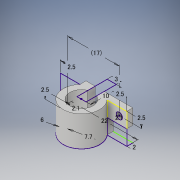
# Autodesk Inventor part: Ω型
Saved by Autodesk Inventor 2019.3 (Build 233278000, 278)
## iProperties
Created: 2019-08-08
Part Number: Ω型
Material: 一般
Document SubType Name: Modeling
Designer: naito
Density: 1 g/cm^3
Appearance: 既定
Author: naito
Autodesk Inventor part; units mm, degrees
ref_plane "YZ Plane" through (0, 0, 0) normal (1, 0, 0) x (0, 1, 0)
ref_plane "XZ Plane" through (0, 0, 0) normal (0, 1, 0) x (-1, 0, 0)
ref_plane "XY Plane" through (0, 0, 0) normal (0, 0, 1) x (1, 0, 0)
sketch "スケッチ3" plane through (0, 0, 0) normal (0, 1, 0) x (-1, 0, 0)
  circle A0 centre (0, 0) radius 3.85
  line L0 (11, -4) -> (4.4721, -4)
  line L1 (-11, -4) -> (-11, -6)
  line L2 (-11, -6) -> (11, -6)
  line L3 (11, -6) -> (11, -4)
  arc A1 (4.4721, -4) -> (-4.4721, -4) centre (0, 0) ccw
  line L4 (-4.4721, -4) -> (-11, -4)
  point P0 (0, -4)
  point P1 (0, -6)
  dimension "d12" = 7.7
  dimension "d14" = 22
  dimension "d15" = 2
  dimension "d16" = 6
  constraints: 10 end point, 3 parallel, 2 centre point, 2 coincident, 2 horizontal, 2 perpendicular, 2 point on circle, 2 vertical alignment, 1 midpoint, 1 point on line
  measures "d12" diameter of A0
  measures "d14" distance of L2.end L1.end
  measures "d15" distance of L1.end L1.start
  measures "d16" radius of A1
extrude "押し出し3" add sketch "スケッチ3" along normal blind 10
sketch "スケッチ4" plane through (4.4721, 0, -4) normal (0, 0, 1) x (1, 0, 0)
  circle A0 centre (4.0279, 7.5) radius 1.05
  circle A1 centre (-12.9721, 2.5) radius 1.05
  line L0 (-15.4721, 0) -> (-15.4721, 10) projected
  line L1 (6.5279, 0) -> (6.5279, 10) projected
  line L2 (0, 10) -> (6.5279, 10) projected
  line L3 (-15.4721, 0) -> (-8.9443, 0) projected
  line L4 (0, 0) -> (0, 10) projected
  line L5 (0, 0) -> (6.5279, 0) projected
  line L6 (0, 0) -> (6.5279, 0) projected
  line L7 (6.5279, 0) -> (6.5279, 10) projected
  line L8 (0, 10) -> (6.5279, 10) projected
  line L9 (0, 0) -> (0, 10) projected
  line L10 (6.5279, 5) -> (0, 5)
  line L11 (0, 0) -> (6.5279, 0) projected
  line L12 (6.5279, 5) -> (6.5279, 0)
  line L13 (6.5279, 0) -> (0, 0)
  line L14 (1.5279, 0) -> (-10.4721, 0) projected
  line L15 (0, 0) -> (0, 5)
  line L16 (-15.4721, 0) -> (-8.9443, 0) projected
  line L17 (-8.9443, 0) -> (-8.9443, 10) projected
  line L18 (-15.4721, 10) -> (-8.9443, 10) projected
  line L19 (-15.4721, 0) -> (-15.4721, 10) projected
  line L20 (-15.4721, 0) -> (-15.4721, 10) projected
  line L21 (-15.4721, 10) -> (-8.9443, 10) projected
  line L22 (-15.4721, 5) -> (-8.9443, 5)
  line L23 (-8.9443, 5) -> (-8.9443, 10)
  line L24 (-8.9443, 10) -> (-15.4721, 10)
  line L25 (-15.4721, 10) -> (-15.4721, 5)
  point P0 (-4.4721, 0)
  dimension "d19" = 2.1
  dimension "d20" = 2.1
  dimension "d21" = 2.5
  dimension "d22" = 2.5
  dimension "d29" = 2.5
  dimension "d30" = 2.5
  dimension "d35" = 17
  constraints: 16 end point, 3 midpoint, 2 centre point, 2 collinear, 2 parallel, 1 horizontal, 1 perpendicular, 1 vertical
  measures "d19" diameter of A0
  measures "d20" diameter of A1
  measures "d21" distance from line of A1.centre L0
  measures "d22" distance from line of A0.centre L1
  measures "d29" distance from line of L2 A0.centre
  measures "d30" distance from line of L3 A1.centre
  measures "d35" horizontal distance of A0.centre A1.centre
extrude "押し出し4" cut sketch "スケッチ4" against normal blind 10 contours A0 | A1
sketch "スケッチ5" plane through (0, 10, 0) normal (0, 1, 0) x (1, 0, 0)
  line L0 (-1.5, 0) -> (1.5, 0)
  line L1 (1.5, 0) -> (1.5, 10)
  line L2 (1.5, 10) -> (-1.5, 10)
  line L3 (-1.5, 10) -> (-1.5, 0)
  point P0 (0, 0)
  point P1 (0, 0)
  dimension "d25" = 3
  dimension "d26" = 10
  constraints: 8 end point, 2 parallel, 1 coincident, 1 horizontal, 1 midpoint, 1 perpendicular
  measures "d25" distance of L2.end L1.end
  measures "d26" distance of L1.end L0.end
extrude "押し出し5" cut sketch "スケッチ5" against normal blind 10
extrude "押し出し6" cut sketch "スケッチ4" against normal blind 2 contours L4 L10 L1 L5
extrude "押し出し7" cut sketch "スケッチ4" against normal blind 2 contours L0 L18 L17 L22
